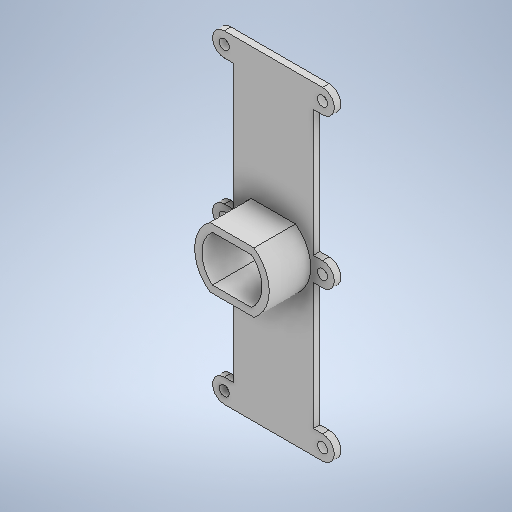
# Autodesk Inventor part: Gripper_MotorHolder
Saved by Autodesk Inventor 2025.1 (Build 291241000, 241)
## iProperties
Created: 2024-08-03
Part Number: Gripper_MotorHolder
Material: Generic
Document SubType Name: Modeling
Designer: leonh
Density: 1 g/cm^3
Appearance: Default
Author: leonh
Autodesk Inventor part; units mm, degrees
ref_plane "YZ Plane" through (0, 0, 0) normal (1, 0, 0) x (0, 1, 0)
ref_plane "XZ Plane" through (0, 0, 0) normal (0, 1, 0) x (-1, 0, 0)
sketch "Sketch1" plane through (0, 0, 0) normal (0, 0, 1) x (1, 0, 0)
  line L0 (-8.124, 9.5) -> (8.124, 9.5)
  line L1 (-8.124, -9.5) -> (8.124, -9.5)
  line L2 (-14.5312, 0) -> (9.3904, 0) construction
  arc A0 (-8.124, 9.5) -> (-8.124, -9.5) centre (0, 0) ccw
  arc A1 (8.124, -9.5) -> (8.124, 9.5) centre (0, 0) ccw
  line L3 (-29.5712, -67.25) -> (29.5712, -67.25)
  line L4 (29.5712, 67.25) -> (-29.5712, 67.25)
  arc A2 (-20.4, -57.45) -> (-20.4, -67.25) centre (-20.4, -62.35) ccw
  line L5 (-20.4, -67.25) -> (-29.5712, -67.25)
  line L6 (-20.4, -57.45) -> (-16.6, -57.45)
  circle A3 centre (-20.4, -62.35) radius 2.1
  line L7 (0, -40.5988) -> (0, 24.1265) construction
  arc A4 (-20.4, 67.25) -> (-20.4, 57.45) centre (-20.4, 62.35) ccw
  line L8 (-20.4, 67.25) -> (-29.5712, 67.25)
  line L9 (-20.4, 57.45) -> (-16.6, 57.45)
  circle A5 centre (-20.4, 62.35) radius 2.1
  arc A6 (20.4, -67.25) -> (20.4, -57.45) centre (20.4, -62.35) ccw
  line L10 (20.4, -67.25) -> (29.5712, -67.25)
  line L11 (20.4, -57.45) -> (16.6, -57.45)
  circle A7 centre (20.4, -62.35) radius 2.1
  line L12 (20.4, 57.45) -> (16.6, 57.45)
  circle A8 centre (20.4, 62.35) radius 2.1
  line L13 (20.4, 67.25) -> (29.5712, 67.25)
  arc A9 (20.4, 57.45) -> (20.4, 67.25) centre (20.4, 62.35) ccw
  arc A10 (-20.4, 4.9) -> (-20.4, -4.9) centre (-20.4, 0) ccw
  line L14 (-20.4, -4.9) -> (-16.6, -4.9)
  line L15 (-20.4, 4.9) -> (-16.6, 4.9)
  circle A11 centre (-20.4, 0) radius 2.1
  line L16 (-16.6, 57.45) -> (-16.6, 4.9)
  line L17 (-16.6, -4.9) -> (-16.6, -57.45)
  line L18 (20.4, 4.9) -> (16.6, 4.9)
  arc A12 (20.4, -4.9) -> (20.4, 4.9) centre (20.4, 0) ccw
  circle A13 centre (20.4, 0) radius 2.1
  line L19 (20.4, -4.9) -> (16.6, -4.9)
  line L20 (16.6, -57.45) -> (16.6, -4.9)
  line L21 (16.6, 4.9) -> (16.6, 57.45)
  line L22 (9.1652, -12.5) -> (-9.1652, -12.5)
  arc A14 (-9.1652, 12.5) -> (-9.1652, -12.5) centre (0, 0) ccw
  line L23 (-9.1652, 12.5) -> (9.1652, 12.5)
  arc A15 (9.1652, -12.5) -> (9.1652, 12.5) centre (0, 0) ccw
  point P0 (-42.7024, 0)
  dimension "d1" = 19
  dimension "d2" = 4.2
  dimension "d3" = 4.9
  dimension "d4" = 134.5
  dimension "d5" = 4.2
  dimension "d6" = 4.9
  dimension "d9" = 3
  dimension "d34" = 33.2
  dimension "d35" = 3.8
  dimension "d36" = 3.8
  dimension "d37" = 12.5
  dimension "d38" = 12.5
  constraints: 48 end point, 24 symmetric about line, 20 point on circle, 16 centre point, 9 coincident, 8 perpendicular, 5 parallel, 4 horizontal, 4 tangent, 3 horizontal alignment, 1 vertical, 12 other
  measures "d1" distance between parallel lines of L1 L0
  measures "d2" diameter of A3
  measures "d3" radius of A2
  measures "d4" distance between parallel lines of L4 L3
  measures "d5" diameter of A11
  measures "d6" radius of A10
  measures "d9" distance between parallel lines of L1 L22
  measures "d34" distance between parallel lines of L21 L16
  measures "d35" distance from line of L21 A9.centre
  measures "d36" distance from line of L21 A13.centre
  measures "d37" radius of A1
  measures "d38" radius of A0
extrude "Extrusion1" add sketch "Sketch1" along normal blind 2.75 contours A2 L6 L17 L14 A10 L15 L16 L9 A4 L4 A9 L12 L21 L18 A12 L19 L20 L11 A6 L3 | L22 A14 L23 A15
extrude "Extrusion2" add sketch "Sketch1" along normal blind 20 contours L22 A14 L23 A15
ref_plane "Work Plane1" through (0, 0, 52.75) normal (0, 0, 1) x (1, 0, 0)
body "Solid1"
